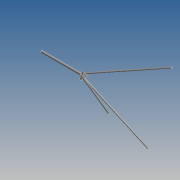
# Autodesk Inventor part: P003_tripod
Saved by Autodesk Inventor 2020 (Build 240168000, 168)
## iProperties
Created: 2021-09-24
Part Number: P003_tripod
Material: Générique
Document SubType Name: Modeling
Designer: gabri
Density: 1 g/cm^3
Appearance: Par défaut
Author: gabri
Autodesk Inventor part; units mm, degrees
sketch "Esquisse2" plane through (0, 0, 0) normal (1, 0, 0) x (0, 1, 0)
  circle A0 centre (0, 0) radius 15
  dimension "d3" = 30
  constraints: 1 centre point, 1 coincident
  measures "d3" diameter of A0
extrude "Extrusion1" add sketch "Esquisse2" along normal blind 600
sketch "Esquisse3" plane through (600, 0, 0) normal (1, 0, 0) x (0, 0, -1)
  circle A0 centre (0, 0) radius 15 construction
  line L0 (35.7678, -45.3211) -> (21.3653, 53.6363)
  line L1 (21.3653, 53.6363) -> (-57.1331, -8.3153)
  line L2 (-57.1331, -8.3153) -> (35.7678, -45.3211)
  line L3 (54.348, 0) -> (-75.7133, 0) construction
  dimension "d12" = 60
  dimension "d13" = 60
  dimension "d14" = 60
  dimension "d16" = 100
  dimension "d17" = 86.6025
  dimension "d18" = 28.8675
  dimension "d19" = 28.8675
  dimension "d20" = 28.8675
  dimension "d21" = 38.281
  constraints: 6 end point
  measures "d12" angle of L1 L0
  measures "d13" angle of L2 L1
  measures "d14" angle of L2 L0
  measures "d16" distance of L0.end L1.end
  measures "d17" distance from line of L0.end L2
  measures "d18" distance from line of L2 A0.centre
  measures "d19" distance from line of L1 A0.centre
  measures "d20" distance from line of A0.centre L0
  measures "d21" angle of L3 L1
extrude "Extrusion2" add sketch "Esquisse3" along normal blind 30
ref_plane "Plan de construction1" through (630, -8.3153, 57.1331) normal (-0.8660254, 0.4645044, -0.1850289) x (0, -0.3700577, -0.9290088)
ref_plane "Plan de construction2" through (630, -45.3211, -35.7678) normal (-0.8660254, -0.0720125, 0.494787) x (0, 0.989574, 0.144025)
ref_plane "Plan de construction3" through (630, 53.6363, -21.3653) normal (-0.8660254, -0.3924919, -0.3097582) x (0, -0.6195163, 0.7849838)
sketch "Esquisse4" plane through (630, -45.3211, -35.7678) normal (-0.8660254, -0.0720125, 0.494787) x (0, 0.989574, 0.144025)
  line L0 (0, 15) -> (100, 15) construction
  line L1 (100, 15) -> (100, 0) construction
  line L2 (0, 0) -> (100, 0) construction
  line L3 (0, 15) -> (0, 0) construction
  circle A0 centre (50, 7.5) radius 10
  line L4 (50, 753.3118) -> (50, -218.5479) construction
  point P0 (50, 290)
  dimension "d25" = 20
  dimension "d26" = 15
  dimension "d27" = 7.5
  constraints: 1 centre point, 1 point on line
  measures "d25" diameter of A0
  measures "d26" distance between parallel lines of L2 L0
  measures "d27" distance from line of A0.centre L0
extrude "Extrusion3" add sketch "Esquisse4" along normal blind 40 and the other way blind 1000
sketch "Esquisse5" plane through (630, 53.6363, -21.3653) normal (-0.8660254, -0.3924919, -0.3097582) x (0, -0.6195163, 0.7849838)
  line L0 (0, 15) -> (100, 15) construction
  line L1 (100, 15) -> (100, 0) construction
  line L2 (0, 0) -> (100, 0) construction
  line L3 (0, 15) -> (0, 0) construction
  circle A0 centre (50, 7.5) radius 10
  line L4 (50, 845.2082) -> (50, -1048.939) construction
  point P0 (50, 290)
  dimension "d32" = 20
  dimension "d33" = 7.5
  constraints: 1 centre point, 1 point on line
  measures "d32" diameter of A0
  measures "d33" distance from line of L0 A0.centre
extrude "Extrusion4" add sketch "Esquisse5" along normal blind 40 and the other way blind 1000
sketch "Esquisse6" plane through (630, -8.3153, 57.1331) normal (-0.8660254, 0.4645044, -0.1850289) x (0, -0.3700577, -0.9290088)
  line L0 (0, 15) -> (100, 15) construction
  line L1 (100, 15) -> (100, 0) construction
  line L2 (0, 0) -> (100, 0) construction
  line L3 (0, 15) -> (0, 0) construction
  circle A0 centre (50, 7.5) radius 10
  line L4 (50, 943.564) -> (50, -1296.7643) construction
  point P0 (50, 290)
  dimension "d38" = 20
  dimension "d39" = 7.5
  constraints: 1 centre point, 1 point on line
  measures "d38" diameter of A0
  measures "d39" distance from line of L0 A0.centre
extrude "Extrusion5" add sketch "Esquisse6" along normal blind 40 and the other way blind 1000
equation "\"d18\" = 0.333333 * d17"
equation "\"d19\" = 0.333333 * d17"
equation "\"d27\" = 0.5 * d26"
